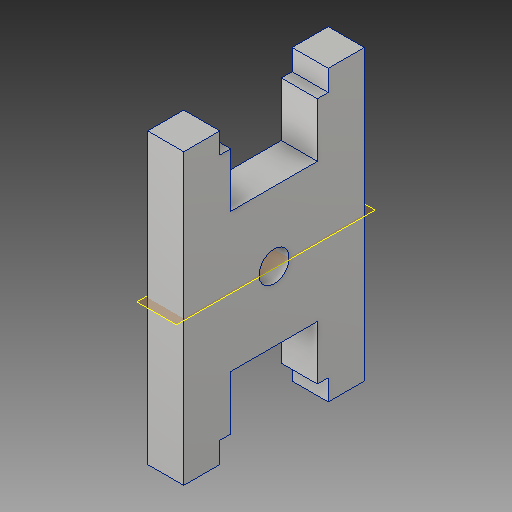
# Autodesk Inventor part: StopMechanismPushPlate
Saved by Autodesk Inventor 2017 (Build 210142000, 142)
## iProperties
Created: 2016-02-17
Part Number: StopMechanismPushPlate
Material: Aluminum 6061
Document SubType Name: Modeling
Designer: steele
Density: 2.7 g/cm^3
Appearance: Aluminum - Flat
Mass: 23.3695 g
Surface Area: 39.9911 cm^2
Volume: 8.65535 cm^3
Author: steele
Autodesk Inventor part; units mm, degrees
ref_plane "YZ Plane" through (0, 0, 0) normal (1, 0, 0) x (0, 1, 0)
ref_plane "XY Plane" through (0, 0, 0) normal (0, 0, 1) x (1, 0, 0)
sketch "Sketch4" plane through (0, 0, 0) normal (1, 0, 0) x (0, 1, 0)
  line L0 (-25.4, 15.875) -> (-25.4, -15.875)
  line L1 (-25.4, -15.875) -> (25.4, -15.875)
  line L2 (25.4, -15.875) -> (25.4, 15.875)
  line L3 (25.4, 15.875) -> (-25.4, 15.875)
  line L4 (-25.4, 15.875) -> (25.4, -15.875) construction
  line L5 (-25.4, -15.875) -> (25.4, 15.875) construction
  point P0 (0, 0)
  dimension "d11" = 50.8
  dimension "d12" = 31.75
  constraints: 12 end point, 2 midpoint, 2 parallel, 1 perpendicular, 1 vertical
  measures "d11" distance of L2.end L0.start
  measures "d12" distance of L0.start L0.end
extrude "Extrusion4" add sketch "Sketch4" along normal blind 6.35
sketch "Sketch5" plane through (0, 0, 0) normal (-1, 0, 0) x (0, 0, 1)
  circle A0 centre (0, 0) radius 2.6543
  dimension "d15" = 5.3086
  constraints: 1 centre point, 1 coincident
  measures "d15" diameter of A0
extrude "Extrusion5" cut sketch "Sketch5" against normal through all
sketch "Sketch7" plane through (6.35, 0, 0) normal (1, 0, 0) x (0, 0, -1)
  line L0 (15.875, 25.4) -> (-15.875, 25.4) projected
  line L1 (-9.525, 25.4) -> (9.525, 25.4)
  line L2 (9.525, 25.4) -> (9.525, 21.717)
  line L3 (9.525, 21.717) -> (-9.525, 21.717)
  line L4 (-9.525, 21.717) -> (-9.525, 25.4)
  line L5 (-15.875, 25.4) -> (-15.875, -25.4) projected
  point P0 (0, 0)
  dimension "d25" = 19.05
  dimension "d26" = 6.35
  dimension "d27" = 3.683
  constraints: 8 end point, 2 parallel, 1 horizontal, 1 perpendicular, 1 point on line
  measures "d25" distance of L2.end L3.end
  measures "d26" distance between parallel lines of L4 L5
  measures "d27" distance between parallel lines of L3 L0
extrude "Extrusion7" cut sketch "Sketch7" against normal through all
mirror "Mirror2" about plane through (0, 0, 0) normal (0, 1, 0) of "Extrusion7"
sketch "Sketch8" plane through (6.35, 0, 0) normal (1, 0, 0) x (0, 0, -1)
  line L0 (0, 12.192) -> (7.62, 12.192)
  line L1 (7.62, 12.192) -> (7.62, 21.717)
  line L2 (7.62, 21.717) -> (-7.62, 21.717)
  line L3 (-7.62, 21.717) -> (-7.62, 12.192)
  line L4 (-7.62, 12.192) -> (0, 12.192)
  line L5 (9.525, 21.717) -> (-9.525, 21.717) projected
  point P0 (0, 0)
  dimension "d30" = 9.525
  dimension "d32" = 7.62
  dimension "d33" = 7.62
  constraints: 10 end point, 3 perpendicular, 2 collinear, 1 horizontal, 1 point on line
  measures "d30" distance between parallel lines of L4 L2
  measures "d32" distance from line of point (0, 0) L3
  measures "d33" distance from line of point (0, 0) L1
extrude "Extrusion8" cut sketch "Sketch8" against normal through all
mirror "Mirror3" about plane through (0, 0, 0) normal (0, 1, 0) of "Extrusion8"
equation "\"d11\" = pushPlateLength"
equation "\"d12\" = pushPlateWidth"
equation "\"stopMechanismWidth\" = 50.8"
equation "\"materialThickness\" = 3.175"
equation "\"stopMechanismLength\" = 50.8"
equation "\"stopMEchamismHeight\" = 50.8"
equation "\"stopMechanismHoleForPost\" = 9.525"
equation "\"pushPlateLength\" = 50.8"
equation "\"pushPlateWidth\" = 31.75"
equation "\"slotWidth\" = 12.7"
equation "\"slotDepth\" = 9.525"
body "Solid2"
